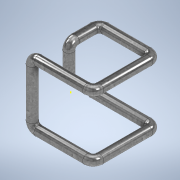
# Autodesk Inventor part: 3D pipe
Saved by Autodesk Inventor 2020 (Build 240168000, 168)
## iProperties
Created: 2021-02-02
Part Number: 3D pipe
Material: Generic
Document SubType Name: Modeling
Designer: Pratishtha  Arya
Density: 1 g/cm^3
Appearance: Steel Galvanized
Author: Pratishtha  Arya
Autodesk Inventor part; units mm, degrees
ref_plane "YZ Plane" through (0, 0, 0) normal (1, 0, 0) x (0, 1, 0)
sketch "Sketch1" plane through (0, 0, 0) normal (1, 0, 0) x (0, 1, 0)
  point P0 (0, 0)
ref_plane "Work Plane1" through (18.1974, 0.6131, -18.949) normal (0, 1, 0) x (-1, 0, 0)
sketch "Sketch2" plane through (18.1974, 0.6131, -18.949) normal (0, 1, 0) x (-1, 0, 0)
  point P0 (18.1974, 18.949)
ref_plane "Work Plane2" through (0, 0.6131, 0) normal (0, 1, 0) x (-1, 0, 0)
ref_plane "Work Plane3" through (18.1974, 0.6131, -18.949) normal (1, 0, 0) x (0, 1, 0)
sketch "Sketch3" plane through (18.1974, 0.6131, -18.949) normal (1, 0, 0) x (0, 1, 0)
  circle A0 centre (0, 0) radius 7.5
  point P0 (-0.6131, 18.949)
  dimension "d17" = 15
  constraints: 1 centre point
  measures "d17" diameter of A0
sketch3d "3D Sketch1"
  line L0 (18.1974, 0.6131, -18.949) -> (108.1974, 0.6131, -18.949)
  arc A0 (108.1974, 0.6131, -18.949) -> (118.1974, 0.6131, -8.949) centre (108.1974, 0.6131, -8.949) ccw
  line L1 (118.1974, 0.6131, -8.949) -> (118.1974, 0.6131, 71.051)
  arc A1 (118.1974, 0.6131, 71.051) -> (108.1974, 0.6131, 81.051) centre (108.1974, 0.6131, 71.051) ccw
  line L2 (108.1974, 0.6131, 81.051) -> (28.1974, 0.6131, 81.051)
  arc A2 (28.1974, 0.6131, 81.051) -> (18.1974, 10.6131, 81.051) centre (28.1974, 10.6131, 81.051) ccw
  line L3 (18.1974, 10.6131, 81.051) -> (18.1974, 90.6131, 81.051)
  arc A3 (18.1974, 90.6131, 81.051) -> (28.1974, 100.6131, 81.051) centre (28.1974, 90.6131, 81.051) ccw
  line L4 (28.1974, 100.6131, 81.051) -> (108.1974, 100.6131, 81.051)
  arc A4 (108.1974, 100.6131, 81.051) -> (118.1974, 100.6131, 71.051) centre (108.1974, 100.6131, 71.051) ccw
  line L5 (118.1974, 100.6131, 71.051) -> (118.1974, 100.6131, -8.949)
  arc A5 (118.1974, 100.6131, -8.949) -> (108.1974, 100.6131, -18.949) centre (108.1974, 100.6131, -8.949) ccw
  line L6 (108.1974, 100.6131, -18.949) -> (38.1974, 100.6131, -18.949)
  arc A6 (38.1974, 100.6131, -18.949) -> (28.1974, 100.6131, -8.949) centre (38.1974, 100.6131, -8.949) ccw
  line L7 (28.1974, 100.6131, -8.949) -> (28.1974, 100.6131, 21.051)
  arc A7 (28.1974, 100.6131, 21.051) -> (28.1974, 90.6131, 31.051) centre (28.1974, 90.6131, 21.051) ccw
  line L8 (28.1974, 90.6131, 31.051) -> (28.1974, 50.6131, 31.051)
  dimension "d0" = 100
  dimension "d1" = 100
  dimension "d2" = 100
  dimension "d3" = 100
  dimension "d4" = 100
  dimension "d5" = 50
  dimension "d6" = 50
  dimension "d7" = 90
  dimension "d8" = 100
  dimension "d9" = 10
  dimension "d10" = 10
  dimension "d11" = 10
  dimension "d12" = 10
  dimension "d13" = 10
  dimension "d14" = 10
  dimension "d15" = 10
  dimension "d16" = 10
sweep "Sweep1" add profiles "Sketch3" path "3D Sketch1"
shell "Shell1" thickness 1.5 removed faces 2 at (18.1974, 2.4843, -17.2912) at (28.7956, 50.6131, 29.7358)
equation "\"d10\" = d9"
equation "\"d11\" = d9"
equation "\"d12\" = d9"
equation "\"d13\" = d9"
equation "\"d14\" = d9"
equation "\"d15\" = d9"
equation "\"d16\" = d9"
body "Solid1"
